Autodesk Inventor part; units mm, degrees
(part 2 of 2)
  line L230 (3.5342, -14.9605) -> (3.5342, -15.1704)
  spline S275 degree 2 poles (3.5342, -15.1704) (3.6597, -15.0449) (3.9067, -14.907) (4.0549, -14.907) knots 0 0 0 1 2 2 2
  spline S276 degree 2 poles (4.0549, -14.907) (4.2237, -14.907) (4.4851, -15.0614) (4.5531, -15.2363) knots 0 0 0 1 2 2 2
  spline S277 degree 2 poles (4.5531, -15.2363) (4.6992, -15.0737) (4.975, -14.907) (5.1356, -14.907) knots 0 0 0 1 2 2 2
  spline S278 degree 2 poles (5.1356, -14.907) (5.2591, -14.907) (5.4608, -14.9831) (5.5349, -15.0696) knots 0 0 0 1 2 2 2
  spline S279 degree 2 poles (5.5349, -15.0696) (5.6111, -15.156) (5.6954, -15.4154) (5.6954, -15.6109) knots 0 0 0 1 2 2 2
  line L231 (5.6954, -15.6109) -> (5.6954, -16.8665)
  line L232 (5.6954, -16.8665) -> (5.3743, -16.8665)
  dimension "d31" = 15.24
  dimension "d32" = 1.27
  dimension "d33" = 3.81
  constraints: 8 end point, 6 horizontal, 2 parallel, 8 other
  measures "d31" distance from line of L0 point (0, 0)
  measures "d32" distance from line of point (0, 0) L2
  measures "d33" distance from line of L3 point (0, 0)
extrude "Extrusion5" cut sketch "Sketch6" against normal blind 1.905
equation "\"d0\" = outerDiameter"
equation "\"d3\" = innerDiameter"
equation "\"d9\" = screwRadius"
equation "\"d10\" = screwRadius"
equation "\"d23\" = allenKeyHole4_0mm"
equation "\"d24\" = allenKeyHole3_5mm"
equation "\"d25\" = allenKeyHole3_0mm"
equation "\"d26\" = allenKeyHole2_5mm"
equation "\"d27\" = allenKeyHole2_0mm"
equation "\"d28\" = allenKeyHold1_5mm"
equation "\"innerDiameter\" = 31.75"
equation "\"edgeRadius\" = 4.699"
equation "\"allenKey3_0mm\" = 3"
equation "\"allenKeyClearance\" = 0.2"
equation "\"allenKeyHole3_0mm\" = allenKey3_0mm + allenKeyClearance"
equation "\"screwRadius\" = 0.5 * innerDiameter + 0.5 * edgeRadius"
equation "\"allenKey4_0mm\" = 4"
equation "\"allenKey3_5mm\" = 3.5"
equation "\"allenKey2_5mm\" = 2.5"
equation "\"alleyKey2_0mm\" = 2"
equation "\"allenKey1_5mm\" = 1.5"
equation "\"allenKeyHole4_0mm\" = allenKey4_0mm + allenKeyClearance"
equation "\"allenKeyHole2_5mm\" = allenKey2_5mm + allenKeyClearance"
equation "\"allenKeyHole2_0mm\" = alleyKey2_0mm + allenKeyClearance"
equation "\"allenKeyHole3_5mm\" = allenKey3_5mm + allenKeyClearance"
equation "\"allenKeyHold1_5mm\" = allenKey1_5mm + allenKeyClearance"
equation "\"outerDiameter\" = 41.148"
body "Solid1"
